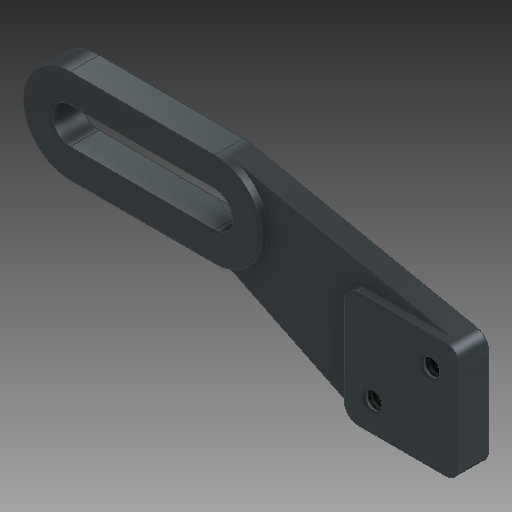
# Autodesk Inventor part: ToolRestarm
Saved by Autodesk Inventor 2020 (Build 240168000, 168)
## iProperties
Created: 2019-11-15
Part Number: ToolRestarm
Material: Iron, Cast
Document SubType Name: Modeling
Designer: Jorge
Density: 7.15 g/cm^3
Appearance: Iron Gray
Author: Jorge
Autodesk Inventor part; units mm, degrees
ref_plane "YZ Plane" through (0, 0, 0) normal (1, 0, 0) x (0, 1, 0)
ref_plane "XZ Plane" through (0, 0, 0) normal (0, 1, 0) x (-1, 0, 0)
ref_plane "XY Plane" through (0, 0, 0) normal (0, 0, 1) x (1, 0, 0)
sketch "Sketch1" plane through (0, 0, 0) normal (0, 0, 1) x (1, 0, 0)
  line L0 (0, 0) -> (31.75, 0) construction
  line L1 (0, -10.3188) -> (28.8982, -10.3188)
  line L2 (31.75, 10.3187) -> (0, 10.3187)
  arc A0 (0, 10.3187) -> (0, -10.3188) centre (0, 0) ccw
  arc A1 (33.8327, 10.1064) -> (31.75, 10.3187) centre (31.75, 0) ccw
  line L3 (85.725, -3.175) -> (85.725, -22.225)
  line L4 (82.55, -25.4) -> (63.5, -25.4)
  line L5 (33.8327, 10.1064) -> (83.1908, -0.0653)
  arc A2 (82.55, -25.4) -> (85.725, -22.225) centre (82.55, -22.225) ccw
  arc A3 (85.725, -3.175) -> (83.1908, -0.0653) centre (82.55, -3.175) ccw
  arc A4 (62.1088, -25.079) -> (63.5, -25.4) centre (63.5, -22.225) ccw
  line L6 (34.463, -11.6028) -> (62.1088, -25.079)
  arc A5 (34.463, -11.6028) -> (28.8982, -10.3188) centre (28.8982, -23.0187) ccw
  point P0 (15.875, 0)
  point P1 (31.8281, -10.3185)
  dimension "d0" = 3.175
  dimension "d1" = 50.8
  dimension "d2" = 31.75
  dimension "d4" = 10.3187
  dimension "d5" = 12.7
  dimension "d6" = 19.05
  dimension "d7" = 3.175
  dimension "d8" = 19.05
  dimension "d9" = 13.0232
  dimension "d10" = 3.175
  dimension "d11" = 154.013
  constraints: 16 end point, 13 point on circle, 13 tangent, 6 centre point, 2 perpendicular, 1 equal radius, 1 horizontal, 1 midpoint, 1 parallel, 1 point on line
  measures "d0" radius of A2
  measures "d1" horizontal distance of A3.centre L0.end
  measures "d2" distance of L0.start L0.end
  measures "d4" radius of A0
  measures "d5" radius of A5
  measures "d6" distance of A2.centre A3.centre
  measures "d7" distance from line of A3.centre L0
  measures "d8" distance of A2.centre A4.centre
  measures "d9" horizontal distance of A5.centre point (15.875, 0)
  measures "d10" distance from line of A2.centre L4
  measures "d11" angle of L4 L6
extrude "Extrusion1" add sketch "Sketch1" along normal blind 4.7625
sketch "Sketch2" plane through (0, 0, 4.7625) normal (0, 0, 1) x (1, 0, 0)
  line L0 (83.1908, -0.0653) -> (33.8327, 10.1064) construction
  arc A0 (33.8327, 10.1064) -> (31.75, 10.3187) centre (31.75, 0) ccw construction
  line L1 (31.75, 10.3187) -> (0, 10.3187) construction
  arc A1 (0, 10.3187) -> (0, -10.3188) centre (0, 0) ccw construction
  line L2 (0, -10.3188) -> (28.8982, -10.3188) construction
  arc A2 (34.463, -11.6028) -> (28.8982, -10.3188) centre (28.8982, -23.0187) ccw construction
  line L3 (34.463, -11.6028) -> (62.1088, -25.079) construction
  arc A3 (62.1088, -25.079) -> (63.5, -25.4) centre (63.5, -22.225) ccw construction
  line L4 (63.5, -25.4) -> (82.55, -25.4) construction
  arc A4 (82.55, -25.4) -> (85.725, -22.225) centre (82.55, -22.225) ccw construction
  line L5 (85.725, -22.225) -> (85.725, -3.175) construction
  arc A5 (85.725, -3.175) -> (83.1908, -0.0653) centre (82.55, -3.175) ccw construction
  line L6 (0, 0) -> (31.75, 0) construction
  line L7 (0, -10.3188) -> (31.75, -10.3188)
  line L8 (31.75, 10.3188) -> (0, 10.3188)
  arc A6 (0, 10.3188) -> (0, -10.3188) centre (0, 0) ccw
  arc A7 (31.75, -10.3188) -> (31.75, 10.3188) centre (31.75, 0) ccw
  point P0 (15.875, 0)
  dimension "d14" = 31.75
  constraints: 8 end point, 4 point on circle, 4 tangent, 2 centre point, 1 concentric, 1 horizontal, 1 midpoint, 1 parallel
  measures "d14" distance of L6.start L6.end
extrude "Extrusion2" add sketch "Sketch2" along normal blind 1.5875
sketch "Sketch3" plane through (0, 0, 0) normal (0, 0, -1) x (-1, 0, 0)
  line L0 (-82.55, -25.4) -> (-63.5, -25.4)
  line L1 (-60.325, -22.225) -> (-60.325, -3.175)
  line L2 (-63.5, 0) -> (-82.55, 0)
  line L3 (-85.725, -3.175) -> (-85.725, -22.225)
  line L4 (-83.1908, -0.0653) -> (-33.8327, 10.1064) construction
  arc A0 (-83.1908, -0.0653) -> (-85.725, -3.175) centre (-82.55, -3.175) ccw construction
  line L5 (-85.725, -22.225) -> (-85.725, -3.175) construction
  arc A1 (-85.725, -22.225) -> (-82.55, -25.4) centre (-82.55, -22.225) ccw construction
  line L6 (-63.5, -25.4) -> (-82.55, -25.4) construction
  arc A2 (-63.5, -25.4) -> (-62.1088, -25.079) centre (-63.5, -22.225) ccw construction
  line L7 (-34.463, -11.6028) -> (-62.1088, -25.079) construction
  arc A3 (-28.8982, -10.3188) -> (-34.463, -11.6028) centre (-28.8982, -23.0187) ccw construction
  line L8 (0, -10.3188) -> (-28.8982, -10.3188) construction
  arc A4 (0, -10.3188) -> (0, 10.3187) centre (0, 0) ccw construction
  line L9 (-31.75, 10.3187) -> (0, 10.3187) construction
  arc A5 (-31.75, 10.3187) -> (-33.8327, 10.1064) centre (-31.75, 0) ccw construction
  arc A6 (-82.55, 0) -> (-85.725, -3.175) centre (-82.55, -3.175) ccw
  arc A7 (-85.725, -22.225) -> (-82.55, -25.4) centre (-82.55, -22.225) ccw
  arc A8 (-63.5, -25.4) -> (-60.325, -22.225) centre (-63.5, -22.225) ccw
  arc A9 (-60.325, -3.175) -> (-63.5, 0) centre (-63.5, -3.175) ccw
  line L10 (-63.5, -25.4) -> (-82.55, -25.4) projected
  point P0 (-60.325, 0)
  point P1 (-60.325, -25.4)
  point P2 (-85.725, 0)
  dimension "d17" = 25.4
  dimension "d18" = 25.4
  dimension "d19" = 3.175
  constraints: 8 end point, 8 point on circle, 8 tangent, 6 point on line, 4 centre point, 3 equal radius, 2 collinear, 2 parallel, 1 horizontal, 1 perpendicular
  measures "d17" distance of point (-85.725, 0) point (-60.325, 0)
  measures "d18" distance of point (-60.325, 0) point (-60.325, -25.4)
  measures "d19" radius of A6
extrude "Extrusion3" add sketch "Sketch3" against normal blind 6.35
sketch "Sketch4" plane through (0, 0, 6.35) normal (0, 0, 1) x (1, 0, 0)
  line L0 (0, -10.3188) -> (31.75, -10.3188) construction
  arc A0 (31.75, -10.3188) -> (31.75, 10.3188) centre (31.75, 0) ccw construction
  line L1 (31.75, 10.3188) -> (0, 10.3188) construction
  arc A1 (0, 10.3188) -> (0, -10.3188) centre (0, 0) ccw construction
  line L2 (0, 0) -> (31.75, 0) construction
  line L3 (0, -3.9688) -> (31.75, -3.9688)
  line L4 (31.75, 3.9688) -> (0, 3.9688)
  arc A2 (0, 3.9688) -> (0, -3.9688) centre (0, 0) ccw
  arc A3 (31.75, -3.9688) -> (31.75, 3.9688) centre (31.75, 0) ccw
  point P0 (15.875, 0)
  dimension "d22" = 7.9375
  constraints: 8 end point, 4 point on circle, 4 tangent, 2 centre point, 1 horizontal, 1 midpoint, 1 parallel
  measures "d22" diameter of A3
extrude "Extrusion4" cut sketch "Sketch4" against normal blind 6.35
sketch "Sketch5" plane through (0, 0, 0) normal (0, 0, -1) x (-1, 0, 0)
  line L0 (-85.725, -22.225) -> (-85.725, -3.175) construction
  line L1 (-63.5, -25.4) -> (-82.55, -25.4) construction
  point P0 (0, 0)
  point P1 (-79.375, -6.35)
  point P2 (-66.675, -19.05)
  dimension "d25" = 19.05
  dimension "d26" = 6.35
  dimension "d27" = 12.7
  dimension "d28" = 6.35
  measures "d25" distance from line of L0 point (-66.675, -19.05)
  measures "d26" distance from line of point (-79.375, -6.35) L0
  measures "d27" horizontal distance of point (-66.675, -19.05) point (-79.375, -6.35)
  measures "d28" distance from line of L1 point (-66.675, -19.05)
hole "Hole1" at (66.675, -19.05, 0) at (79.375, -6.35, 0) direction (0, 0, 1) diameter 3.683 end through all countersink diameter 10.3188 countersink angle 82 thread size "10-24 UNC" class "2B" standard "ANSI Unified Screw Threads"
equation "\"d8\" = d6"
body "Solid1"
